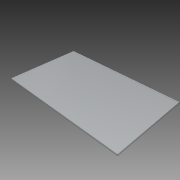
# Autodesk Inventor part: protect_plexi
Saved by Autodesk Inventor 2014 (Build 180170000, 170)
## iProperties
Created: 2013-12-12
Part Number: protect_plexi
Material: Glass
Document SubType Name: Modeling
Designer: buben
Density: 2.18 g/cm^3
Appearance: Clear
Author: buben
Autodesk Inventor part; units mm, degrees
ref_plane "YZ Plane" through (0, 0, 0) normal (1, 0, 0) x (0, 1, 0)
ref_plane "XZ Plane" through (0, 0, 0) normal (0, 1, 0) x (-1, 0, 0)
ref_plane "XY Plane" through (0, 0, 0) normal (0, 0, 1) x (1, 0, 0)
sketch "Sketch1" plane through (0, 0, 0) normal (0, 0, 1) x (1, 0, 0)
  line L0 (0, 0) -> (239, 0)
  line L1 (239, 0) -> (239, 145)
  line L2 (239, 145) -> (0, 145)
  line L3 (0, 145) -> (0, 0)
  dimension "d0" = 239
  dimension "d1" = 145
  constraints: 8 end point, 2 parallel, 1 horizontal, 1 perpendicular
  measures "d0" distance of L0.start L0.end
  measures "d1" distance of L2.end L0.start
extrude "Extrusion1" add sketch "Sketch1" along normal blind 3
chamfer "Chamfer1" distance 0.5 angle 45 12 edges at (0, 72.5, 3) (119.5, 145, 3) (119.5, 0, 3) (239, 72.5, 3) (119.5, 0, 0) (239, 72.5, 0) (119.5, 145, 0) (0, 72.5, 0) (0, 0, 1.5) (0, 145, 1.5) (239, 0, 1.5) (239, 145, 1.5)
body "Solid1"
